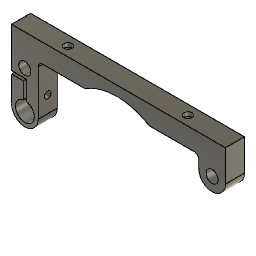
JRCNC0016 v16 (Autodesk Fusion 360 design; units mm, degrees)
Autodesk Fusion 360 part; units mm, degrees
sketch "Sketch1" plane through (0, 0, 0) normal (0, 0, 1) x (1, 0, 0)
  line L0 (71.4, 6.35) -> (-71.4, 6.35)
  line L1 (-71.4, 6.35) -> (-71.4, -6.35)
  line L2 (-71.4, -6.35) -> (71.4, -6.35)
  line L3 (71.4, -6.35) -> (71.4, 6.35)
  line L4 (71.4, 6.35) -> (-71.4, -6.35) construction
  line L5 (-71.4, 6.35) -> (71.4, -6.35) construction
  dimension "d1" = 142.8
  dimension "d2" = 12.7
  constraint horizontal L0
  constraint perpendicular L0 L1
  constraint parallel L0 L2
  constraint parallel L1 L3
  constraint coincident L4 origin
  constraint coincident L5 origin
  measures "d1" distance of L0.start L0.end
  measures "d2" distance of L0.start L2.end
extrude "Extrude1" add sketch "Sketch1" along normal blind 12.7
sketch "Sketch2" plane through (0, 6.35, 0) normal (0, 1, 0) x (-1, 0, 0)
  line L0 (-71.4, 0) -> (71.4, 0)
  line L1 (71.4, 0) -> (71.4, 12.7)
  line L2 (71.4, 12.7) -> (-71.4, 12.7)
  line L3 (-71.4, 12.7) -> (-71.4, 0)
  circle A0 centre (-62.51, -8.3) radius 8.89
  circle A1 centre (62.51, -8.3) radius 8.89
  line L4 (-62.51, -8.3) -> (62.51, -8.3) construction
  line L5 (0, 0) -> (0, -8.3) construction
  line L6 (-71.4, -8.3) -> (-53.62, -8.3)
  line L7 (-53.62, -8.3) -> (-53.62, 12.7)
  line L8 (-53.62, 12.7) -> (-71.4, 12.7)
  line L9 (-71.4, 12.7) -> (-71.4, -8.3)
  line L10 (71.4, -8.3) -> (53.62, -8.3)
  line L11 (53.62, -8.3) -> (53.62, 12.7)
  line L12 (53.62, 12.7) -> (71.4, 12.7)
  line L13 (71.4, 12.7) -> (71.4, -8.3)
  dimension "d6" = 17.78
  dimension "d7" = 17.78
  dimension "d19" = 21
  constraint coincident A0.centre L4.start
  constraint parallel L0 L4
  constraint coincident A1.centre L4.end
  constraint coincident L5.start origin
  constraint perpendicular L0 L5
  constraint midpoint L4 L5.end
  constraint horizontal L6
  constraint vertical L7
  constraint horizontal L8
  constraint vertical L9
  constraint coincident A0 L6.start
  constraint horizontal L10
  constraint vertical L11
  constraint horizontal L12
  constraint vertical L13
  constraint coincident L2 L11.end
  constraint coincident A1 L10.start
  constraint coincident A1 L10.end
  constraint coincident L4 L10.end
  constraint coincident A0 L6.end
  constraint coincident L4 L6.end
  constraint coincident L2.end L3.start
  measures "d6" diameter of A0
  measures "d7" diameter of A1
  measures "d19" distance of A1.centre L12
extrude "Extrude2" add sketch "Sketch2" against normal blind 12.7 contours L0 L2 L3 A0 L7 L8 L9 | L0 A0 L9 | L0 A0 | L0 A0 L6 | A0 L6 | L0 A0 L7 | L0 L1 L2 A1 L11 L12 L13 | L0 A1 L11 | L0 A1 | L0 A1 L10 | A1 L10 | L0 A1 L13
sketch "Sketch3" plane through (0, -6.35, 0) normal (0, -1, 0) x (1, 0, 0)
  line L0 (-53.62, 0) -> (53.62, 0)
  line L1 (53.62, 0) -> (53.62, -8.3)
  arc A0 (53.62, -8.3) -> (71.4, -8.3) centre (62.51, -8.3) ccw
  line L2 (71.4, -8.3) -> (71.4, 12.7)
  line L3 (71.4, 12.7) -> (-71.4, 12.7)
  line L4 (-71.4, 12.7) -> (-71.4, -8.3)
  arc A1 (-71.4, -8.3) -> (-53.62, -8.3) centre (-62.51, -8.3) ccw
  line L5 (-53.62, -8.3) -> (-53.62, 0)
  circle A2 centre (-62.51, -8.3) radius 4.0625
  circle A3 centre (62.51, -8.3) radius 4.0625
  dimension "d11" = 8.125
  dimension "d12" = 8.125
  constraint concentric A1 A2
  constraint concentric A0 A3
  measures "d11" diameter of A3
  measures "d12" diameter of A2
extrude "Extrude3" cut sketch "Sketch3" against normal blind 10 contours A2 | A3
sketch "Sketch4" plane through (0, 0, 0) normal (0, 0, -1) x (1, 0, 0)
  line L0 (-53.62, 6.35) -> (-53.62, -6.35)
  line L1 (-53.62, -6.35) -> (53.62, -6.35)
  line L2 (53.62, -6.35) -> (53.62, 6.35)
  line L3 (53.62, 6.35) -> (-53.62, 6.35)
  line L4 (-40, 0) -> (40, 0)
  dimension "d15" = 80
  constraint parallel L3 L4
  constraint midpoint origin L4
  measures "d15" distance of L4.start L4.end
hole "Hole1" at (-40, 0, 0) at (40, 0, 0) direction (0, 0, 1) diameter 5.5 depth 35 tip angle 180 counterbore diameter 10 counterbore depth 10
sketch "Sketch5" plane through (0, 6.35, 0) normal (0, 1, 0) x (-1, 0, 0)
  line L0 (71.4, 12.7) -> (-71.4, 12.7)
  line L1 (-71.4, 12.7) -> (-71.4, -8.3)
  arc A0 (-71.4, -8.3) -> (-53.62, -8.3) centre (-62.51, -8.3) ccw
  line L2 (-53.62, -8.3) -> (-53.62, 0)
  line L3 (-53.62, 0) -> (53.62, 0)
  line L4 (53.62, 0) -> (53.62, -8.3)
  arc A1 (53.62, -8.3) -> (71.4, -8.3) centre (62.51, -8.3) ccw
  line L5 (71.4, -8.3) -> (71.4, 12.7)
  circle A2 centre (62.51, -33.3) radius 8.89
  line L6 (62.51, -8.3) -> (62.51, -33.3)
  line L7 (53.62, -8.3) -> (71.4, -8.3)
  line L8 (71.4, -8.3) -> (71.4, -33.3)
  line L9 (71.4, -33.3) -> (53.62, -33.3)
  line L10 (53.62, -33.3) -> (53.62, -8.3)
  circle A3 centre (62.51, -33.3) radius 6.3
  dimension "d20" = 25
  dimension "d21" = 12.6
  constraint coincident A1.centre L6.start
  constraint coincident A2.centre L6.end
  constraint perpendicular L3 L6
  constraint horizontal L7
  constraint vertical L8
  constraint horizontal L9
  constraint vertical L10
  constraint coincident A2 L8.end
  constraint coincident L4.end A1.start
  constraint coincident A1.end L5.start
  constraint coincident A2.centre L9
  constraint concentric A2 A3
  measures "d20" distance of A1.centre A2.centre
  measures "d21" diameter of A3
extrude "Extrude4" add sketch "Sketch5" against normal blind 12.7 contours A1 A2 L6 L8 | A1 A2 L6 L10 | A2 L6 L9 A3 | A2 L9 A3 | A2 L6 L9 A3
fillet "Fillet1" radius 3 2 edges at (-53.62, 0, 0) (53.62, 0, 0)
sketch "Sketch6" plane through (0, 0, 12.7) normal (0, 0, 1) x (-1, 0, 0)
  circle A0 centre (40, 0) radius 2.75
  circle A1 centre (-40, 0) radius 2.75
  line L0 (71.4, 6.35) -> (-71.4, 6.35)
  line L1 (-71.4, 6.35) -> (-71.4, -6.35)
  line L2 (-71.4, -6.35) -> (71.4, -6.35)
  line L3 (71.4, -6.35) -> (71.4, 6.35)
  line L4 (62.5, -6.35) -> (-62.5, -6.35)
  line L5 (-62.5, -6.35) -> (-62.5, 6.35)
  line L6 (-62.5, 6.35) -> (62.5, 6.35)
  line L7 (62.5, 6.35) -> (62.5, -6.35)
  line L8 (62.5, -6.35) -> (-62.5, 6.35) construction
  line L9 (-62.5, -6.35) -> (62.5, 6.35) construction
  dimension "d26" = 125
  constraint horizontal L4
  constraint perpendicular L4 L5
  constraint parallel L4 L6
  constraint parallel L5 L7
  constraint coincident L2 L4.start
  constraint coincident L8 origin
  constraint coincident L9 origin
  measures "d26" distance of L4.start L4.end
sketch "Sketch7" plane through (0, 6.35, 0) normal (0, 1, 0) x (-1, 0, 0)
  circle A0 centre (62.51, -33.3) radius 6.3
  line L0 (71.4, 12.7) -> (-71.4, 12.7)
  line L1 (-71.4, 12.7) -> (-71.4, -8.3)
  arc A1 (-71.4, -8.3) -> (-53.62, -8.3) centre (-62.51, -8.3) ccw
  line L2 (-53.62, -8.3) -> (-53.62, -3)
  arc A2 (-50.62, 0) -> (-53.62, -3) centre (-50.62, -3) ccw
  line L3 (-50.62, 0) -> (50.62, 0)
  arc A3 (53.62, -3) -> (50.62, 0) centre (50.62, -3) ccw
  line L4 (53.62, -3) -> (53.62, -33.3)
  arc A4 (53.62, -33.3) -> (71.4, -33.3) centre (62.51, -33.3) ccw
  line L5 (71.4, -33.3) -> (71.4, 12.7)
  line L6 (61.51, -27.0799) -> (63.51, -27.0799)
  line L7 (63.51, -27.0799) -> (63.51, -14.0799)
  line L8 (63.51, -14.0799) -> (61.51, -14.0799)
  line L9 (61.51, -14.0799) -> (61.51, -27.0799)
  line L10 (61.51, -27.0799) -> (63.51, -14.0799) construction
  line L11 (63.51, -27.0799) -> (61.51, -14.0799) construction
  line L12 (63.51, -14.0799) -> (71.4, -14.0799)
  line L13 (71.4, -14.0799) -> (71.4, -16.0799)
  line L14 (71.4, -16.0799) -> (63.51, -16.0799)
  line L15 (63.51, -16.0799) -> (63.51, -14.0799)
  line L16 (63.51, -14.0799) -> (71.4, -16.0799) construction
  line L17 (71.4, -14.0799) -> (63.51, -16.0799) construction
  line L18 (62.51, -33.3) -> (62.51, 32.4202) construction
  point P0 (62.51, -20.5799)
  point P1 (67.455, -15.0799)
  point P2 (62.51, -27.0799)
  dimension "d29" = 2
  dimension "d30" = 2
  dimension "d31" = 13
  constraint horizontal L6
  constraint perpendicular L6 L7
  constraint parallel L6 L8
  constraint parallel L7 L9
  constraint coincident A0 L6.start
  constraint coincident L10 P0
  constraint coincident L11 P0
  constraint horizontal L12
  constraint perpendicular L12 L13
  constraint parallel L12 L14
  constraint parallel L13 L15
  constraint coincident L16 P1
  constraint coincident L17 P1
  constraint coincident L5 L13.end
  constraint coincident A0.centre A4.centre
  constraint vertical L18
  constraint midpoint L6 P2
  constraint coincident L18 P2
  measures "d29" distance of L8 L13.end
  measures "d30" distance of L7.end L8.end
  measures "d31" distance of L6.end L7.end
extrude "Extrude6" cut sketch "Sketch7" against normal blind 21 contours A0 L7 L8 L9 L15 | L5 L7 L12 L13 L14 L15
sketch "Sketch8" plane through (-71.4, 0, 0) normal (-1, 0, 0) x (0, -1, 0)
  line L0 (6.35, -16.0799) -> (-6.35, -16.0799)
  line L1 (-6.35, -16.0799) -> (-6.35, -33.3)
  line L2 (-6.35, -33.3) -> (6.35, -33.3)
  line L3 (6.35, -33.3) -> (6.35, -16.0799)
  line L4 (-6.35, -16.0799) -> (6.35, -16.0799)
  line L5 (6.35, -16.0799) -> (6.35, -28.7799)
  line L6 (6.35, -28.7799) -> (-6.35, -28.7799)
  line L7 (-6.35, -28.7799) -> (-6.35, -16.0799)
  line L8 (-6.35, -16.0799) -> (6.35, -28.7799) construction
  line L9 (6.35, -16.0799) -> (-6.35, -28.7799) construction
  point P0 (0, -22.4299)
  constraint horizontal L4
  constraint perpendicular L4 L5
  constraint parallel L4 L6
  constraint parallel L5 L7
  constraint coincident L0.end L1.start
  constraint coincident L8 P0
  constraint coincident L9 P0
  constraint equal L4 L7
  constraint coincident L3 L5.end
hole "Hole2" at (-71.4, 0, -22.4299) direction (1, 0, 0) diameter 3.9 depth 22 tip angle 118
hole "Hole3" at (-53.62, 0, -22.4299) direction (-1, 0, 0) diameter 4.496 depth 4 tip angle 118
sketch "Sketch9" plane through (0, -6.35, 0) normal (0, -1, 0) x (1, 0, 0)
  line L0 (-63.51, -16.0799) -> (-71.4, -16.0799)
  line L1 (-71.4, -16.0799) -> (-71.4, -33.3)
  arc A0 (-71.4, -33.3) -> (-53.62, -33.3) centre (-62.51, -33.3) ccw
  line L2 (-53.62, -33.3) -> (-53.62, -3)
  arc A1 (-50.62, 0) -> (-53.62, -3) centre (-50.62, -3) ccw
  line L3 (-50.62, 0) -> (50.62, 0)
  arc A2 (53.62, -3) -> (50.62, 0) centre (50.62, -3) ccw
  line L4 (53.62, -3) -> (53.62, -8.3)
  arc A3 (53.62, -8.3) -> (71.4, -8.3) centre (62.51, -8.3) ccw
  line L5 (71.4, -8.3) -> (71.4, 12.7)
  line L6 (71.4, 12.7) -> (-71.4, 12.7)
  line L7 (-71.4, 12.7) -> (-71.4, -14.0799)
  line L8 (-71.4, -14.0799) -> (-61.51, -14.0799)
  line L9 (-61.51, -14.0799) -> (-61.51, -27.0799)
  arc A4 (-63.51, -27.0799) -> (-61.51, -27.0799) centre (-62.51, -33.3) ccw
  line L10 (-63.51, -27.0799) -> (-63.51, -16.0799)
  circle A5 centre (-62.51, -8.3) radius 4.0625
  circle A6 centre (62.51, -8.3) radius 4.0625
  line L11 (-0.9045, 12.7) -> (-0.9045, -33.8)
  circle A7 centre (-0.9045, -33.8) radius 40
  dimension "d42" = 46.5
  dimension "d43" = 80
  constraint coincident L6 L11.start
  constraint perpendicular L6 L11
  constraint coincident L11.end A7.centre
  measures "d42" distance of L11.start L11.end
  measures "d43" diameter of A7
extrude "Extrude7" cut sketch "Sketch9" against normal blind 19 contours L3 L11 A7 | L3 L11 A7
equation "d42 = 51 mm - 4.5 mm"
